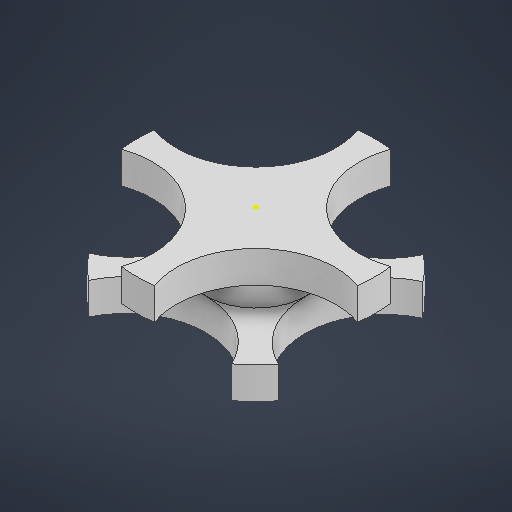
# Autodesk Inventor part: Part1
Saved by Autodesk Inventor 2026 (Build 300175000, 175)
## iProperties
Created: 2025-10-14
Part Number: Part1
Material: 一般
Document SubType Name: Modeling
Designer: masak
Density: 1 g/cm^3
Appearance: 既定
Author: masak
Autodesk Inventor part; units mm, degrees
ref_plane "YZ Plane" through (0, 0, 0) normal (1, 0, 0) x (0, 1, 0)
ref_plane "XZ Plane" through (0, 0, 0) normal (0, 1, 0) x (-1, 0, 0)
ref_plane "XY Plane" through (0, 0, 0) normal (0, 0, 1) x (1, 0, 0)
sketch "スケッチ1" plane through (0, 0, 0) normal (0, 1, 0) x (-1, 0, 0)
  circle A0 centre (0, 0) radius 25
  circle A1 centre (0, 0) radius 30
  dimension "d0" = 50
  dimension "d1" = 60
  constraints: 2 centre point, 2 coincident
  measures "d0" diameter of A0
  measures "d1" diameter of A1
extrude "押し出し1" add sketch "スケッチ1" along normal blind 8 contours A0 | A1
sketch "スケッチ2" plane through (0, 8, 0) normal (0, 1, 0) x (1, 0, 0)
  circle A0 centre (0, 0) radius 30 projected
  line L0 (0, -30) -> (-30, 0)
  line L1 (-30, 0) -> (0, 30)
  line L2 (0, 30) -> (30, 0)
  line L3 (0, -30) -> (30, 0)
  circle A1 centre (0, 0) radius 30
  circle A2 centre (0, 0) radius 25
  circle A3 centre (-23, 23) radius 20
  circle A4 centre (-23, -23) radius 20
  circle A5 centre (23, -23) radius 20
  circle A6 centre (23, 23) radius 20
  point P0 (-4.1593, 29.7103)
  point P1 (-29.7103, 4.1593)
  dimension "d5" = 50
  dimension "d8" = 23
  dimension "d9" = 23
  dimension "d13" = 360
  dimension "d29" = 40
  constraints: 8 end point, 6 centre point, 3 point on circle, 2 coincident, 1 concentric, 9 other
  measures "d5" diameter of A2
  measures "d8" horizontal distance of A3.centre point (0, 0)
  measures "d9" horizontal distance of point (0, 0) A3.centre
  measures "d29" diameter of A3
extrude "押し出し2" cut sketch "スケッチ2" against normal blind 10 contours A6 L2 A2 A0 | A0 A6 | A5 A0 | A0 A5 L3 A2 | A6 A2 L2 | L3 A2 A5 | A2 A6 L2 | L2 A2 | A2 L3 | L3 A2 A5 | L2 A2 A6 | A5 A2 L3 | A3 L1 A2 A0 | A0 A3 | A3 A2 L1 | A4 A0 | A0 A4 L0 A2 | L0 A2 A4 | A3 A2 L1 | A2 L0 A4 | L1 A2 | A2 L0 | L1 A2 A3 | A4 A2 L0
sketch "スケッチ3" plane through (0, 8, 0) normal (0, 1, 0) x (1, 0, 0)
  point P0 (0, 0)
sketch "スケッチ4" plane through (0, 0, 0) normal (0, -1, 0) x (1, 0, 0)
  circle A0 centre (0, 0) radius 12.5
  dimension "d15" = 25
  constraints: 1 centre point, 1 coincident
  measures "d15" diameter of A0
extrude "押し出し3" add sketch "スケッチ4" along normal blind 5
sketch "スケッチ5" plane through (0, -5, 0) normal (0, -1, 0) x (1, 0, 0)
  circle A0 centre (0, 0) radius 30
  dimension "d18" = 60
  constraints: 1 centre point, 1 coincident
  measures "d18" diameter of A0
extrude "押し出し4" add sketch "スケッチ5" along normal blind 8
sketch "スケッチ6" plane through (0, -13, 0) normal (0, -1, 0) x (1, 0, 0)
  circle A0 centre (-0.2145, 32.5024) radius 20
  circle A1 centre (-32.51, -0.2559) radius 20
  circle A2 centre (0.2483, -32.5514) radius 20
  circle A3 centre (32.5438, 0.2069) radius 20
  point P0 (0.0169, -0.0245)
  point P1 (0.0169, -0.0245)
  point P2 (-3.3011, 29.5474)
  point P3 (-30.0758, 2.7727)
  dimension "d30" = 40
  dimension "d37" = 360
  dimension "d40" = 32.5269
  constraints: 4 centre point, 1 coincident, 9 other
  measures "d30" diameter of A0
  measures "d40" vertical distance of point (0.017, -0.025) A0.centre
extrude "押し出し5" cut sketch "スケッチ6" against normal blind 8
